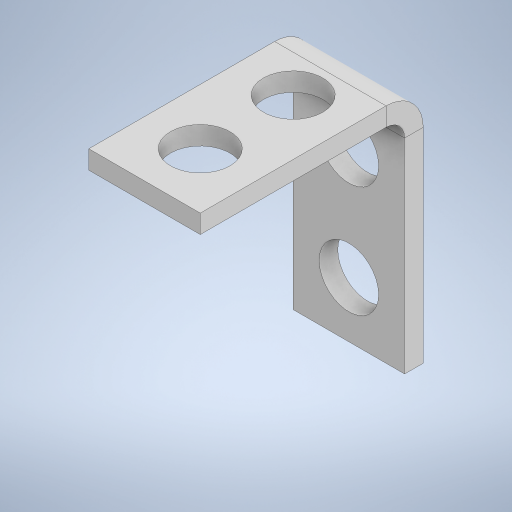
# Autodesk Inventor part: connector_Zshape
Saved by Autodesk Inventor 2023 (Build 270158000, 158)
## iProperties
Created: 2023-06-13
Part Number: connector_Zshape
Material: 一般
Document SubType Name: Sheet Metal
Designer: 310611102
Density: 1 g/cm^3
Sheet Metal Rule: Default_mm
Appearance: 預設
Author: 310611102
Autodesk Inventor part; units mm, degrees
ref_plane "YZ Plane" through (0, 0, 0) normal (1, 0, 0) x (0, 1, 0)
ref_plane "XZ Plane" through (0, 0, 0) normal (0, 1, 0) x (-1, 0, 0)
ref_plane "XY Plane" through (0, 0, 0) normal (0, 0, 1) x (1, 0, 0)
sketch "Sketch1" plane through (0, 0, 0) normal (0, 0, 1) x (1, 0, 0)
  line L0 (-3, 6) -> (3, 6)
  line L1 (3, 6) -> (3, -6)
  line L2 (3, -6) -> (-3, -6)
  line L3 (-3, -6) -> (-3, 6)
  line L4 (-3, 6) -> (3, -6) construction
  line L5 (3, 6) -> (-3, -6) construction
  circle A0 centre (0, 3) radius 1.6
  circle A1 centre (0, -3) radius 1.6
  point P0 (0, 0)
  dimension "d0" = 12
  dimension "d1" = 6
  dimension "d2" = 3.2
  dimension "d3" = 3.2
  dimension "d4" = 6
  dimension "d5" = 3
  measures "d0" distance of L0.end L1.end
  measures "d1" distance of L0.start L0.end
  measures "d2" diameter of A0
  measures "d3" diameter of A1
  measures "d4" distance of A0.centre A1.centre
  measures "d5" distance from line of L2 A1.centre
extrude "Plate1" add sketch "Sketch1" along normal blind 1
sketch "Sketch2" plane through (-3, 6, 1) normal (0, 1, 0) x (-1, 0, 0)
  line L0 (-6, 0) -> (0, 0)
  line L1 (0, 0) -> (0, 11)
  line L2 (0, 11) -> (-6, 11)
  line L3 (-6, 11) -> (-6, 0)
  constraints: 6 end point, 1 horizontal, 1 perpendicular, 1 vertical
edge flange "Flange1" height 12 angle 90 thickness 1 bend radius 1 thickness toward (0, 1, 0) relief straight relief width 1 relief depth 0.5 edges at (0, 6, 1) wall of the first edge with corners at (3, 6, 1) (-3, 6, 1) (-3, 6, 12) (3, 6, 12)
bend "Bend1"
corner "Corner1"
sketch "Sketch5" plane through (-3, 6, 12) normal (0, -1, 0) x (1, 0, 0)
  circle A0 centre (3, -8) radius 1.6
  circle A1 centre (3, -3) radius 1.6
  line L0 (6, 0) -> (0, 0) projected
  point P0 (3, -12)
  point P1 (3, 0)
  dimension "d33" = 3.2
  dimension "d34" = 3.2
  dimension "d35" = 5
  dimension "d36" = 3
  constraints: 2 centre point, 2 vertical alignment, 1 midpoint
  measures "d33" diameter of A0
  measures "d34" diameter of A1
  measures "d35" distance of A1.centre A0.centre
  measures "d36" distance from line of L0 A1.centre
extrude "Cut2" cut sketch "Sketch5" against normal blind 1
equation "\"d37\" = 厚度"
equation "\"d6\" = 厚度"
equation "\"d7\" = 折彎離隙寬度"
equation "\"d8\" = 折彎離隙深度"
equation "\"d9\" = 最小剩餘"
equation "\"d10\" = 轉移半徑"
equation "\"d13\" = 折彎半徑"
equation "\"d14\" = 轉角離隙大小"
equation "\"d15\" = 間隙大小"
equation "\"d16\" = Jacobi半徑大小"
equation "\"折彎半徑\" = 厚度"
equation "\"折彎離隙寬度\" = 厚度"
equation "\"折彎離隙深度\" = 0.5 * 厚度"
equation "\"轉角離隙大小\" = 4 * 厚度"
equation "\"最小剩餘\" = 2 * 厚度"
equation "\"轉移半徑\" = 折彎半徑"
equation "\"Jacobi半徑大小\" = 折彎半徑"
equation "\"間隙大小\" = 厚度"
equation "\"厚度\" = 1"
body "Solid1"
